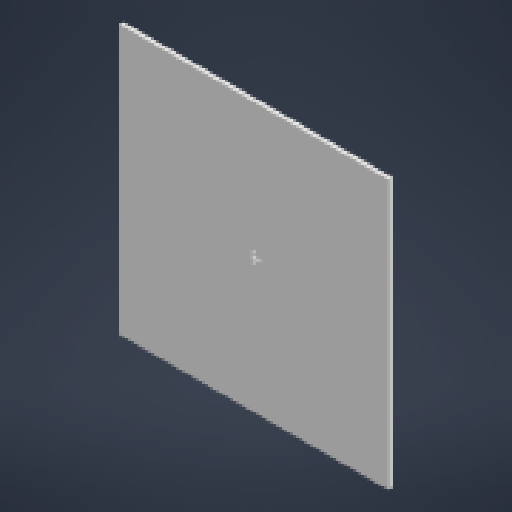
# Autodesk Inventor part: Lasercutplade
Saved by Autodesk Inventor 2026.1 (Build 301233020, 233B)
## iProperties
Created: 2025-12-03
Part Number: Lasercutplade
Material: Generic
Document SubType Name: Modeling
Designer: Mikke
Density: 1 g/cm^3
Appearance: Default
Author: Mikke
Autodesk Inventor part; units mm, degrees
ref_plane "YZ Plane" through (0, 0, 0) normal (1, 0, 0) x (0, 1, 0)
ref_plane "XZ Plane" through (0, 0, 0) normal (0, 1, 0) x (-1, 0, 0)
ref_plane "XY Plane" through (0, 0, 0) normal (0, 0, 1) x (1, 0, 0)
sketch "Sketch1" plane through (0, 0, 0) normal (0, 0, 1) x (1, 0, 0)
  line L0 (-200, 200) -> (200, 200)
  line L1 (200, 200) -> (200, -200)
  line L2 (200, -200) -> (-200, -200)
  line L3 (-200, -200) -> (-200, 200)
  line L4 (-200, 200) -> (200, -200) construction
  line L5 (200, 200) -> (-200, -200) construction
  point P0 (0, 0)
  dimension "d0" = 400
  dimension "d1" = 400
  constraints: 12 end point, 2 midpoint, 2 parallel, 1 horizontal, 1 perpendicular
  measures "d0" distance of L1.end L2.end
  measures "d1" distance of L0.end L1.end
extrude "Extrusion1" add sketch "Sketch1" along normal blind 6
sketch "Sketch2" plane through (0, 0, 6) normal (0, 0, 1) x (1, 0, 0)
  arc A0 (-2.9, -2.0149) -> (-2.9, 2.0149) centre (-0.35, 0) ccw projected
  line L0 (-2.9, 2.0149) -> (-2.9, -2.0149) projected
  circle A1 centre (-0.35, -6.75) radius 2 projected
  circle A2 centre (6.4, 0) radius 2 projected
  circle A3 centre (-0.35, 6.75) radius 2 projected
  circle A4 centre (6.4, 0) radius 2.2
  circle A5 centre (-0.35, 6.75) radius 2.2
  circle A6 centre (-0.35, -6.75) radius 2.2
  arc A7 (-3, -2.0494) -> (-3, 2.0494) centre (-0.35, 0) ccw
  line L1 (-3, -2.0494) -> (-3, 2.0494)
  point P0 (0, 0)
  dimension "d4" = 0.2
  dimension "d5" = 0.2
  dimension "d6" = 0.2
  dimension "d7" = 0.1
  constraints: 4 centre point, 2 end point, 2 point on circle, 1 other
  measures "d4" radial gap between concentric circles of A2 A4
  measures "d5" radial gap between concentric circles of A3 A5
  measures "d6" radial gap between concentric circles of A1 A6
  measures "d7" radial gap between concentric circles of A0 A7
extrude "Extrusion2" cut sketch "Sketch2" against normal blind 6 contours L0 A0 | A1 | A2 | A3 | A4 | A5 | A6 | L1 A7
body "Solid1"
